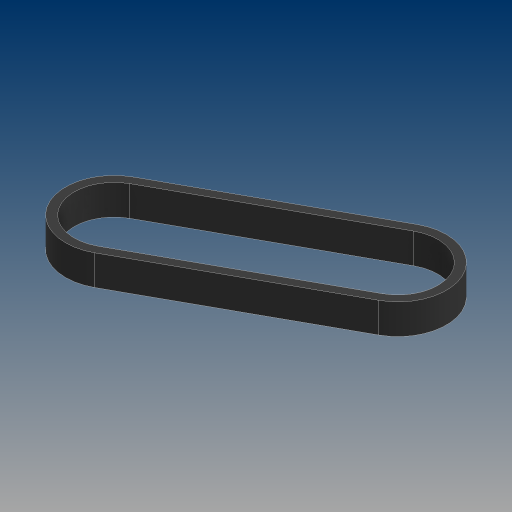
# Autodesk Inventor part: INtk_010_Belt2
Saved by Autodesk Inventor 2024.3 (Build 283343000, 343)
## iProperties
Created: 2024-08-07
Part Number: INtk_010_Belt2
Material: Rubber, Silicone
Document SubType Name: Modeling
Designer: Kenji
Density: 1.25 g/cm^3
Appearance: Rubber - Black
Author: Kenji
Autodesk Inventor part; units mm, degrees
ref_plane "YZ Plane" through (0, 0, 0) normal (1, 0, 0) x (0, 1, 0)
ref_plane "XZ Plane" through (0, 0, 0) normal (0, 1, 0) x (-1, 0, 0)
ref_plane "XY Plane" through (0, 0, 0) normal (0, 0, 1) x (1, 0, 0)
sketch "Sketch1" plane through (0, 0, 0) normal (0, 1, 0) x (-1, 0, 0)
  circle A0 centre (0, 0) radius 11.938 construction
  line L0 (0, 0) -> (-54.7943, -30.1916) construction
  line L1 (0, 0) -> (-11.938, 0) construction
  circle A1 centre (-54.7943, -30.1916) radius 11.938 construction
  line L2 (-49.0331, -40.6475) -> (5.7612, -10.4559)
  line L3 (-60.5554, -19.7358) -> (-5.7612, 10.4559)
  arc A2 (-60.5554, -19.7358) -> (-49.0331, -40.6475) centre (-54.7943, -30.1916) ccw
  arc A3 (5.7612, -10.4559) -> (-5.7612, 10.4559) centre (0, 0) ccw
  line L4 (-6.9869, 12.6805) -> (-61.7812, -17.5111)
  arc A4 (-61.7812, -17.5111) -> (-47.8073, -42.8721) centre (-54.7943, -30.1916) ccw
  line L5 (-47.8073, -42.8721) -> (6.9869, -12.6805)
  arc A5 (6.9869, -12.6805) -> (-6.9869, 12.6805) centre (0, 0) ccw
  dimension "d11" = 23.876
  dimension "d12" = 28.855
  dimension "d13" = 62.5615
  dimension "d14" = 2.54
  constraints: 13 point on circle, 12 end point, 7 tangent, 6 centre point, 3 coincident, 1 equal radius, 1 horizontal, 4 other
  measures "d11" diameter of A0
  measures "d12" angle of L0 L1
  measures "d13" distance of L0.start L0.end
  measures "d14" distance between parallel lines of L3 L4
extrude "Extrusion2" add sketch "Sketch1" along normal blind 8.9916
body "Solid2"
